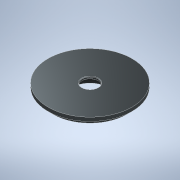
# Autodesk Inventor part: Крышка перегородки11
Saved by Autodesk Inventor 2021 (Build 250183000, 183)
## iProperties
Created: 2020-11-17
Part Number: Крышка перегородки11
Material: Чугун, литейный
Document SubType Name: Modeling
Designer: Тимоха
Density: 7.15 g/cm^3
Appearance: Чугун серый
Mass: 18596.7 g
Surface Area: 2550.69 cm^2
Volume: 2600.94 cm^3
Author: Тимоха
Autodesk Inventor part; units mm, degrees
ref_plane "YZ Plane" through (0, 0, 0) normal (1, 0, 0) x (0, 1, 0)
ref_plane "XZ Plane" through (0, 0, 0) normal (0, 1, 0) x (-1, 0, 0)
ref_plane "XY Plane" through (0, 0, 0) normal (0, 0, 1) x (1, 0, 0)
sketch "Эскиз1" plane through (0, 0, 0) normal (0, 0, 1) x (1, 0, 0)
  line L0 (0, 0) -> (170, 0)
  line L1 (170, 0) -> (170, -15)
  line L2 (170, -15) -> (150, -15)
  line L3 (150, -15) -> (150, -35)
  line L4 (150, -35) -> (110, -35)
  line L5 (110, -35) -> (110, -42.5)
  line L6 (110, -42.5) -> (100, -42.5)
  line L7 (100, -42.5) -> (100, -50)
  line L8 (100, -50) -> (70, -50)
  line L9 (70, -50) -> (70, -10)
  line L10 (70, -10) -> (32, -10)
  line L11 (32, -10) -> (32, 0)
  line L12 (0, 0) -> (0, -18.1999)
  line L13 (150, -20) -> (145, -20)
  line L14 (145, -20) -> (145, -25)
  line L15 (145, -25) -> (150, -25)
  dimension "d0" = 170
  dimension "d1" = 15
  dimension "d2" = 20
  dimension "d3" = 20
  dimension "d4" = 40
  dimension "d5" = 7.5
  dimension "d6" = 10
  dimension "d7" = 7.5
  dimension "d8" = 30
  dimension "d9" = 40
  dimension "d10" = 38
  dimension "d11" = 5
  dimension "d12" = 5
  dimension "d15" = 5
  constraints: 32 end point, 12 perpendicular, 2 horizontal, 2 point on line, 2 vertical, 1 midpoint
  measures "d0" distance of L0.start L0.end
  measures "d1" distance of L0.end L1.end
  measures "d2" distance of L1.end L2.end
  measures "d3" distance of L2.end L3.end
  measures "d4" distance of L3.end L4.end
  measures "d5" distance of L4.end L5.end
  measures "d6" distance of L5.end L6.end
  measures "d7" distance of L6.end L7.end
  measures "d8" distance of L7.end L8.end
  measures "d9" distance of L8.end L9.end
  measures "d10" distance of L9.end L10.end
  measures "d11" distance of L13.start L13.end
  measures "d12" distance of L13.end L14.end
  measures "d15" distance between parallel lines of L13 L2
revolve "Вращение1" add sketch "Эскиз1" angle 360 about axis through (0, 0, 0) along (0, -1, 0) contours L0 L1 L2 L3 L13 L14 L15 L4 L5 L6 L7 L8 L9 L10 L11
fillet "Сопряжение1" radius 2 1 edges at (-100, -42.5, 0)
sketch "Эскиз2" plane through (0, -35, 0) normal (0, -1, 0) x (1, 0, 0)
  circle A0 centre (0, 0) radius 110 projected
  line L0 (0, 0) -> (49.7488, -120.1043)
  line L1 (0, -238) -> (0, 238) projected
  dimension "d16" = 130
  dimension "d17" = 22.5
  constraints: 2 end point
  measures "d16" distance of L0.start L0.end
  measures "d17" angle of L1 L0
hole "Отверстие1" at (49.7488, -35, -120.1043) direction (0, 1, 0) diameter 8 depth 15 tip angle 118 counterbore diameter 12 counterbore depth 10
pattern_circular "Круговой массив1" count 8 over 360 about axis through (0, -30, 0) along (0, -1, 0) of "Отверстие1"
thread "Резьба1" size "M12x1.75" class "6H" standard "ANSI Metric M Profile" full length
thread "Резьба2" size "M12x1.75" class "6H" standard "ANSI Metric M Profile" full length
thread "Резьба3" size "M12x1.75" class "6H" standard "ANSI Metric M Profile" full length
thread "Резьба4" size "M12x1.75" class "6H" standard "ANSI Metric M Profile" full length
thread "Резьба5" size "M12x1.75" class "6H" standard "ANSI Metric M Profile" full length
thread "Резьба6" size "M12x1.75" class "6H" standard "ANSI Metric M Profile" full length
thread "Резьба7" size "M12x1.75" class "6H" standard "ANSI Metric M Profile" full length
thread "Резьба8" size "M12x1.75" class "6H" standard "ANSI Metric M Profile" full length
sketch "Эскиз3" plane through (0, -50, 0) normal (0, -1, 0) x (1, 0, 0)
  circle A0 centre (0, 0) radius 70 projected
  line L0 (0, 0) -> (32.5281, -78.5298)
  line L1 (0, -238) -> (0, 238) projected
  dimension "d44" = 85
  dimension "d45" = 22.5
  constraints: 2 end point
  measures "d44" distance of L0.start L0.end
  measures "d45" angle of L1 L0
hole "Отверстие2" at (32.5281, -50, -78.5298) direction (0, 1, 0) diameter 8 depth 15 tip angle 118 counterbore diameter 12 counterbore depth 10
pattern_circular "Круговой массив2" count 8 over 360 about axis through (0, -30, 0) along (0, -1, 0) of "Отверстие2"
thread "Резьба9" size "M12x1.75" class "6H" standard "ANSI Metric M Profile" full length
thread "Резьба10" size "M12x1.75" class "6H" standard "ANSI Metric M Profile" full length
thread "Резьба11" size "M12x1.75" class "6H" standard "ANSI Metric M Profile" full length
thread "Резьба12" size "M12x1.75" class "6H" standard "ANSI Metric M Profile" full length
thread "Резьба13" size "M12x1.75" class "6H" standard "ANSI Metric M Profile" full length
thread "Резьба14" size "M12x1.75" class "6H" standard "ANSI Metric M Profile" full length
thread "Резьба15" size "M12x1.75" class "6H" standard "ANSI Metric M Profile" full length
thread "Резьба16" size "M12x1.75" class "6H" standard "ANSI Metric M Profile" full length
chamfer "Фаска1" distance 2 angle 45 2 edges at (-32, 0, 0) (-32, -10, 0)
chamfer "Фаска2" distance 2 angle 45 1 edges at (-100, -50, 0)
